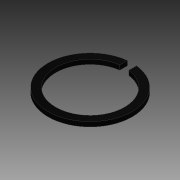
# Autodesk Inventor part: LedHolder
Saved by Autodesk Inventor 2014 (Build 180170000, 170)
## iProperties
Created: 2013-12-17
Part Number: LedHolder
Material: Generic
Document SubType Name: Modeling
Designer: blacki
Density: 1 g/cm^3
Appearance: Plywood - New
Author: blacki
Autodesk Inventor part; units mm, degrees
ref_plane "YZ Plane" through (0, 0, 0) normal (1, 0, 0) x (0, 1, 0)
ref_plane "XZ Plane" through (0, 0, 0) normal (0, 1, 0) x (-1, 0, 0)
ref_plane "XY Plane" through (0, 0, 0) normal (0, 0, 1) x (1, 0, 0)
sketch "Sketch1" plane through (0, 0, 0) normal (0, 0, 1) x (1, 0, 0)
  circle A0 centre (0, 0) radius 27.5
  dimension "d0" = 55
  constraints: 1 centre point, 1 coincident
  measures "d0" diameter of A0
extrude "Extrusion1" add sketch "Sketch1" along normal blind 3
sketch "Sketch2" plane through (0, 0, 3) normal (0, 0, 1) x (1, 0, 0)
  circle A0 centre (0, 0) radius 27.5 projected
  circle A1 centre (0, 0) radius 22.5
  line L0 (-3, 27.5) -> (3, 27.5)
  line L1 (3, 27.5) -> (3, 0)
  line L2 (3, 0) -> (-3, 0)
  line L3 (-3, 0) -> (-3, 27.5)
  line L4 (0, 0) -> (0, 42.337) construction
  point P0 (0, 27.5)
  dimension "d3" = 45
  dimension "d4" = 6
  constraints: 10 end point, 3 parallel, 2 midpoint, 1 centre point, 1 horizontal, 1 perpendicular, 1 point on line, 1 tangent
  measures "d3" diameter of A1
  measures "d4" distance between parallel lines of L1 L3
extrude "Extrusion2" cut sketch "Sketch2" against normal up to next contours L1 A1 L3 A0 | A0 L0 L1 | L3 L0 A0 | L1 L2 L3 A1 | A1 L3 L2 L1 picked at (0, 24.1518)
body "Solid1"
